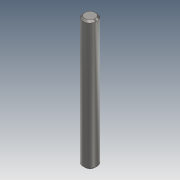
# Autodesk Inventor part: contra-eixo
Saved by Autodesk Inventor 2017 (Build 210142000, 142)
## iProperties
Created: 2018-08-05
Part Number: contra-eixo
Material: Stainless Steel
Document SubType Name: Modeling
Designer: Luiz Gustavo
Density: 8 g/cm^3
Appearance: Semi-Polished
Author: Luiz Gustavo
Autodesk Inventor part; units mm, degrees
ref_plane "YZ Plane" through (0, 0, 0) normal (1, 0, 0) x (0, 1, 0)
ref_plane "XZ Plane" through (0, 0, 0) normal (0, 1, 0) x (-1, 0, 0)
ref_plane "XY Plane" through (0, 0, 0) normal (0, 0, 1) x (1, 0, 0)
sketch "Sketch1" plane through (0, 0, 0) normal (0, 0, 1) x (1, 0, 0)
  circle A0 centre (0, 0) radius 4
  dimension "d0" = 8
  constraints: 1 centre point, 1 coincident
  measures "d0" diameter of A0
extrude "Extrusion1" add sketch "Sketch1" along normal mid plane 75
chamfer "Chamfer1" distance 1 angle 45 2 edges at (-4, 0, 37.5) (-4, 0, -37.5)
body "Solid1"
